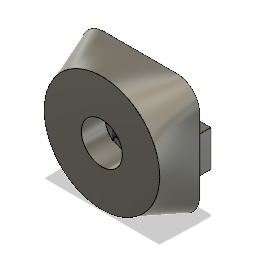
Rigid_feet_for_MK3 (Autodesk Fusion 360 design; units mm, degrees)
Autodesk Fusion 360 part; units mm, degrees
sketch "Sketch1" plane through (0, 0, 0) normal (0, 0, 1) x (1, 0, 0)
  line L0 (5, 0) -> (21, 0)
  line L1 (26, -5) -> (26, -21)
  line L2 (21, -26) -> (5, -26)
  line L3 (0, -21) -> (0, -5)
  arc A0 (5, 0) -> (0, -5) centre (5, -5) ccw
  arc A1 (26, -5) -> (21, 0) centre (21, -5) ccw
  arc A2 (21, -26) -> (26, -21) centre (21, -21) ccw
  arc A3 (0, -21) -> (5, -26) centre (5, -21) ccw
  line L4 (26, -13) -> (0, -13) construction
  line L5 (13, 0) -> (13, -26) construction
  line L6 (-2, -9) -> (-2, -17)
  line L7 (-2, -17) -> (28, -17)
  line L8 (28, -17) -> (28, -9)
  line L9 (28, -9) -> (-2, -17) construction
  line L10 (-2, -9) -> (28, -17) construction
  line L11 (17.5, -9) -> (8.5, -9)
  line L12 (8.5, -9) -> (8.5, -17)
  line L13 (8.5, -17) -> (17.5, -17)
  line L14 (17.5, -17) -> (17.5, -9)
  line L15 (28, -9) -> (-2, -9)
  line L16 (17.5, -9) -> (8.5, -17) construction
  line L17 (8.5, -9) -> (17.5, -17) construction
  dimension "d1" = 26
  dimension "d2" = 26
  dimension "d3" = 5
  dimension "d7" = 30
  dimension "d8" = 8
  dimension "d9" = 9
  dimension "d10" = 8
  measures "d3" radius of A0
ref_plane "WorkPlane1" through (13, -13, 8.5) normal (0, 0, 1) x (1, 0, 0)
sketch "Sketch2" plane through (13, -13, 8.5) normal (0, 0, 1) x (1, 0, 0)
  circle A0 centre (0, 0) radius 12.7
  circle A1 centre (0, 0) radius 4.5
  circle A2 centre (0, 0) radius 2.75
  dimension "d5" = 25.4
  dimension "d13" = 9
  dimension "d14" = 5.5
  measures "d5" diameter of A0
  measures "d13" diameter of A1
  measures "d14" diameter of A2
loft "Loft1" add profiles "Sketch1", "Sketch2" section 1 contours L0 L1 L3 A0 A1 L11 L15 | L3 L7 L12 L15 | L1 L7 L14 L15 | L1 L2 L3 A2 A3 L7 L13 | L7 L11 L12 L13 L14 L15 section 2 contours A0 | A1 | A2
extrude "Extrude1" add sketch "Sketch1" against normal blind 3 contours L3 L7 L12 L15 | L1 L7 L14 L15
extrude "Extrude2" cut sketch "Sketch2" against normal blind 57 contours A2
extrude "Extrude3" cut sketch "Sketch2" against normal blind 5.6 contours A1
sketch "Sketch3" plane through (13, -13, 8.5) normal (0, 0, 1) x (1, 0, 0)
  line L0 (2.75, -6.4761) -> (-2.75, -6.4761)
  line L1 (-2.75, -6.4761) -> (-2.75, 6.4761)
  line L2 (-2.75, 6.4761) -> (2.75, 6.4761)
  line L3 (2.75, 6.4761) -> (2.75, -6.4761)
  line L4 (2.75, -6.4761) -> (-2.75, 6.4761) construction
  line L5 (-2.75, -6.4761) -> (2.75, 6.4761) construction
  line L6 (2.75, 6.4761) -> (5.7962, 6.4761)
  line L7 (5.7962, 6.4761) -> (5.7962, -6.6524)
  line L8 (5.7962, -6.6524) -> (2.75, -6.6524)
  line L9 (2.75, -6.6524) -> (2.75, 6.4761)
  line L10 (-2.75, 6.4761) -> (-6.6744, 6.4761)
  line L11 (-6.6744, 6.4761) -> (-6.6744, -6.6524)
  line L12 (-6.6744, -6.6524) -> (-2.75, -6.6524)
  line L13 (-2.75, -6.6524) -> (-2.75, 6.4761)
  circle A0 centre (0, 0) radius 4.5
  line L14 (10, -2.75) -> (-10, -2.75)
  line L15 (-10, -2.75) -> (-10, 2.75)
  line L16 (-10, 2.75) -> (10, 2.75)
  line L17 (10, 2.75) -> (10, -2.75)
  line L18 (10, -2.75) -> (-10, 2.75) construction
  line L19 (-10, -2.75) -> (10, 2.75) construction
  line L20 (-10, 2.75) -> (10, 2.75)
  line L21 (10, 2.75) -> (10, 8)
  line L22 (10, 8) -> (-10, 8)
  line L23 (-10, 8) -> (-10, 2.75)
  line L24 (-10, -2.75) -> (10, -2.75)
  line L25 (10, -2.75) -> (10, -9)
  line L26 (10, -9) -> (-10, -9)
  line L27 (-10, -9) -> (-10, -2.75)
  dimension "d19" = 5.5
  dimension "d23" = 5.5
extrude "Extrude4" add sketch "Sketch3" along normal blind 0.2 from surface at -5.6 contours L1 L3 L9 L13 A0 L14 L24 | L3 L9 A0 L14 L24 | L1 L13 A0 L14 L24 | L3 L9 A0 L14 L16 L20 L24 | L1 L13 A0 L14 L16 L20 L24 | L1 L3 L9 L13 A0 L16 L20 | L3 L9 A0 L16 L20 | L1 L13 A0 L16 L20
extrude "Extrude5" add sketch "Sketch3" along normal blind 0.2 from surface at -5.4 contours L3 L9 A0 L14 L24 | L1 L13 A0 L14 L24 | L3 L9 A0 L14 L16 L20 L24 | L1 L13 A0 L14 L16 L20 L24 | L3 L9 A0 L16 L20 | L1 L13 A0 L16 L20
chamfer "Chamfer4" distance 0.5 angle 45 8 edges at (26, -13, -3) (21.75, -9, -3) (21.75, -17, -3) (17.5, -13, -3) (8.5, -13, -3) (4.25, -9, -3) (4.25, -17, -3) (0, -13, -3)
equation "d4 = 10.5 mm - 2 mm"
